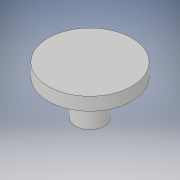
# Autodesk Inventor part: Grabber Base
Saved by Autodesk Inventor 2019.4 (Build 234330000, 330)
## iProperties
Created: 2020-12-03
Part Number: Grabber Base
Material: Generic
Document SubType Name: Modeling
Designer: caleb
Density: 1 g/cm^3
Appearance: Default
Author: caleb
Autodesk Inventor part; units mm, degrees
ref_plane "YZ Plane" through (0, 0, 0) normal (1, 0, 0) x (0, 1, 0)
ref_plane "XZ Plane" through (0, 0, 0) normal (0, 1, 0) x (-1, 0, 0)
ref_plane "XY Plane" through (0, 0, 0) normal (0, 0, 1) x (1, 0, 0)
sketch "Sketch1" plane through (0, 0, 0) normal (0, 1, 0) x (-1, 0, 0)
  circle A0 centre (0, 0) radius 25.98
  dimension "d0" = 51.96
  constraints: 1 centre point, 1 coincident
  measures "d0" diameter of A0
extrude "Extrusion1" add sketch "Sketch1" along normal blind 9.97
sketch "Sketch4" plane through (0, 0, 0) normal (0, -1, 0) x (1, 0, 0)
  circle A0 centre (0, 0) radius 22.21
  circle A1 centre (0, 0) radius 25.98 projected
  dimension "d18" = 44.42
  constraints: 1 centre point, 1 coincident
  measures "d18" diameter of A0
extrude "Extrusion3" cut sketch "Sketch4" against normal blind 1.91
sketch "Sketch6" plane through (0, 0, 0) normal (0, -1, 0) x (1, 0, 0)
  circle A0 centre (0, 0) radius 19
  circle A1 centre (-19, 0) radius 1.525
  circle A2 centre (9.5, -16.4545) radius 1.525
  circle A3 centre (9.5, 16.4545) radius 1.525
  dimension "d21" = 38
  dimension "d22" = 3.05
  dimension "d24" = 19
  dimension "d27" = 360
  constraints: 3 centre point, 1 coincident, 1 horizontal alignment, 9 other
  measures "d22" diameter of A1
  measures "d24" distance of point (0, 0) A1.centre
hole "Hole2" at (-19, 0, 0) at (9.5, 0, 16.4545) at (9.5, 0, -16.4545) direction (0, 1, 0) diameter 3.05 depth 5 tip angle 118
sketch "Sketch7" plane through (0, 0, 0) normal (0, -1, 0) x (1, 0, 0)
  circle A0 centre (0, 0) radius 9
  dimension "d36" = 18
  constraints: 1 centre point, 1 coincident
  measures "d36" diameter of A0
extrude "Extrusion4" add sketch "Sketch7" along normal blind 20.03
sketch "Sketch8" plane through (0, -20.03, 0) normal (0, -1, 0) x (1, 0, 0)
  circle A0 centre (-4, -4) radius 1.5
  circle A1 centre (4, -4) radius 1.5
  circle A2 centre (4, 4) radius 1.5
  circle A3 centre (-4, 4) radius 1.5
  point P0 (0, 0)
  dimension "d39" = 3
  dimension "d40" = 4
  dimension "d41" = 4
  dimension "d44" = 360
  constraints: 4 centre point, 9 other
  measures "d39" diameter of A0
  measures "d40" horizontal distance of point (0, 0) A0.centre
  measures "d41" horizontal distance of point (0, 0) A0.centre
hole "Hole3" at (4, -20.03, -4) at (-4, -20.03, -4) at (-4, -20.03, 4) at (4, -20.03, 4) direction (0, 1, 0) diameter 2.459 depth 8.8 tip angle 118 thread size "M3x0.5" class "6H" standard "ANSI Metric M Profile"
body "Solid1"
